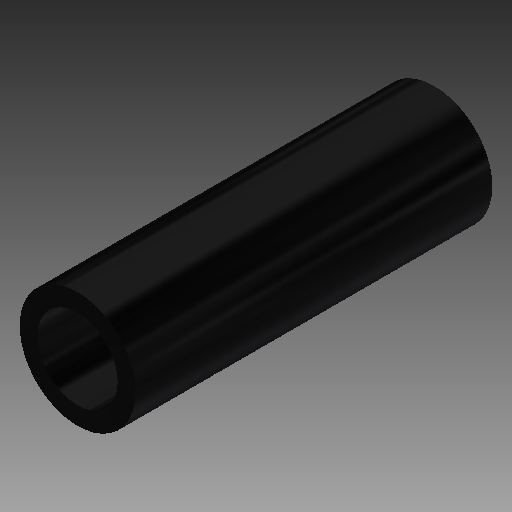
# Autodesk Inventor part: 202-16
Saved by Autodesk Inventor 2019 (Build 230136000, 136)
## iProperties
Company: Autodesk Inc.
Created: 2007-11-04
Part Number: 202-16
Document SubType Name: Modeling
Designer: Autodesk Inc.
Density: 1.425 g/cm^3
Mass: 0.492445 g
Surface Area: 7.25708 cm^2
Volume: 0.345575 cm^3
Material: Acetal Resin, Black
Description: WIRE CONNECTING TUBE
Appearance: Glossy - Black
Component Category: Fasteners
Author: Inventor
Autodesk Inventor part; units mm, degrees
ref_plane "YZ Plane" through (0, 0, 0) normal (1, 0, 0) x (0, 1, 0)
ref_plane "XZ Plane" through (0, 0, 0) normal (0, 1, 0) x (-1, 0, 0)
ref_plane "XY Plane" through (0, 0, 0) normal (0, 0, 1) x (1, 0, 0)
sketch "Sketch1" plane through (0, 0, 0) normal (0, 0, 1) x (1, 0, 0)
  circle A0 centre (0, 0) radius 3.25
  circle A1 centre (0, 0) radius 2.25
  dimension "d0" = 4.5
  dimension "d1" = 6.5
  constraints: 2 centre point, 2 coincident
  measures "d0" diameter of A1
  measures "d1" diameter of A0
extrude "Extrusion1" add sketch "Sketch1" along normal mid plane 20
body "Solid1"
